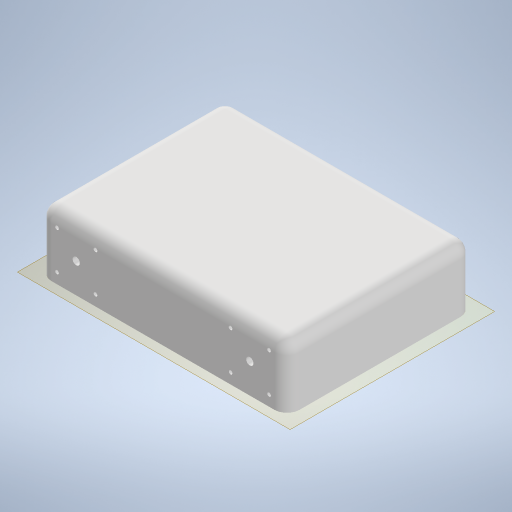
# Autodesk Inventor part: podvozje
Saved by Autodesk Inventor 2024 (Build 280153000, 153)
## iProperties
Created: 2023-09-14
Part Number: podvozje
Material: Generic
Document SubType Name: Modeling
Designer: jebes windows
Density: 1 g/cm^3
Appearance: Default
Author: jebes windows
Autodesk Inventor part; units mm, degrees
ref_plane "YZ Plane" through (0, 0, 0) normal (1, 0, 0) x (0, 1, 0)
ref_plane "XZ Plane" through (0, 0, 0) normal (0, 1, 0) x (-1, 0, 0)
ref_plane "XY Plane" through (0, 0, 0) normal (0, 0, 1) x (1, 0, 0)
ref_plane "Work Plane1" through (0, 0, 0) normal (0, 0, 1) x (1, 0, 0)
sketch "Sketch1" plane through (0, 0, 0) normal (0, 0, 1) x (1, 0, 0)
  line L0 (-90, -75) -> (90, -75) projected
  line L1 (100, -65) -> (100, 65) projected
  line L2 (90, 75) -> (-90, 75) projected
  line L3 (-100, 65) -> (-100, -65) projected
  line L4 (95, 70) -> (95, -70)
  line L5 (95, -70) -> (-95, -70)
  line L6 (-95, -70) -> (-95, 70)
  line L7 (-95, 70) -> (95, 70)
  arc A0 (100, 65) -> (90, 75) centre (90, 65) ccw projected
  arc A1 (-90, 75) -> (-100, 65) centre (-90, 65) ccw projected
  arc A2 (-100, -65) -> (-90, -75) centre (-90, -65) ccw projected
  arc A3 (90, -75) -> (100, -65) centre (90, -65) ccw projected
  point P0 (0, 0)
  dimension "d0" = 5
  constraints: 8 end point, 3 other
  measures "d0" distance between parallel lines of L1 L4
extrude "Extrusion1" add sketch "Sketch1" along normal blind 45
sketch "Sketch2" plane through (0, 0, 45) normal (0, 0, 1) x (1, 0, 0)
  line L0 (-90, -75) -> (90, -75) projected
  line L1 (100, -65) -> (100, 65) projected
  line L2 (90, 75) -> (-90, 75) projected
  line L3 (-100, 65) -> (-100, -65) projected
  line L4 (-90, -75) -> (90, -75) projected
  line L5 (95, 70) -> (95, -70) projected
  line L6 (95, -70) -> (-95, -70) projected
  line L7 (-95, -70) -> (-95, 70) projected
  line L8 (-95, 70) -> (95, 70) projected
  arc A0 (90, -75) -> (100, -65) centre (90, -65) ccw projected
  arc A1 (100, 65) -> (90, 75) centre (90, 65) ccw projected
  arc A2 (-90, 75) -> (-100, 65) centre (-90, 65) ccw projected
  arc A3 (-100, -65) -> (-90, -75) centre (-90, -65) ccw projected
  point P0 (0, 0)
  point P1 (-100, -75)
  point P2 (100, -75)
  point P3 (-100, -75)
  point P4 (100, -75)
extrude "Extrusion2" add sketch "Sketch2" along normal blind 5 contours A3 L3 A2 L2 A1 L1 A0 L0 | L5 L6 L7 L8
sketch "Sketch3" plane through (-95, -70, 0) normal (0, 1, 0) x (1, 0, 0)
  line L0 (180.5, -39.5) -> (149.5, -39.5)
  line L1 (149.5, -39.5) -> (149.5, -8.5)
  line L2 (149.5, -8.5) -> (180.5, -8.5)
  line L3 (180.5, -8.5) -> (180.5, -39.5)
  line L4 (180.5, -39.5) -> (149.5, -8.5) construction
  line L5 (149.5, -39.5) -> (180.5, -8.5) construction
  line L6 (5, 0) -> (185, 0) projected
  line L7 (5, -50) -> (185, -50) projected
  circle A0 centre (149.5, -39.5) radius 1.5
  circle A1 centre (180.5, -39.5) radius 1.5
  circle A2 centre (180.5, -8.5) radius 1.5
  circle A3 centre (149.5, -8.5) radius 1.5
  circle A4 centre (165, -24) radius 3
  line L8 (195, 0) -> (195, -50) projected
  point P0 (95, 0)
  point P1 (-5, 0)
  point P2 (-5, -50)
  dimension "d5" = 31
  dimension "d6" = 31
  dimension "d9" = 10.5
  dimension "d10" = 3
  dimension "d11" = 3
  dimension "d12" = 3
  dimension "d13" = 3
  dimension "d16" = 6
  dimension "d18" = 30
  constraints: 12 end point, 5 centre point, 5 coincident, 2 midpoint, 2 parallel, 1 horizontal, 1 perpendicular
  measures "d5" distance of L1.end L2.end
  measures "d6" distance of L0.end L1.end
  measures "d9" distance between parallel lines of L0 L7
  measures "d10" diameter of A0
  measures "d11" diameter of A1
  measures "d12" diameter of A2
  measures "d13" diameter of A3
  measures "d16" diameter of A4
  measures "d18" distance from line of L8 A4.centre
extrude "Extrusion3" cut sketch "Sketch3" against normal blind 5 contours A0 L1 L0 | L0 L1 A0 | A1 L3 L0 | L0 L3 A1 | A3 L2 L1 | L1 L2 A3 | A2 L2 L3 | L3 L2 A2 | A4
mirror "Mirror1" about plane through (0, 0, 0) normal (1, 0, 0) of "Extrusion3"
mirror "Mirror2" about plane through (0, 0, 0) normal (0, 1, 0) of "Extrusion3"
mirror "Mirror3" about plane through (0, 0, 0) normal (0, 1, 0) of "Extrusion3", "Mirror1"
fillet "Fillet1" radius 10 4 edges at (100, 0, 50) (0, -75, 50) (-100, 0, 50) (0, 75, 50)
body "Solid1"
